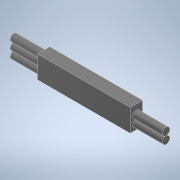
# Autodesk Inventor part: ESC
Saved by Autodesk Inventor 2022 (Build 260153000, 153)
## iProperties
Created: 2022-08-09
Part Number: ESC
Material: Generic
Document SubType Name: Modeling
Designer: Nick
Density: 3.22028 g/cm^3
Appearance: Smooth - Black
Mass: 6.8 g
Surface Area: 17.0549 cm^2
Volume: 2.11162 cm^3
Author: Nick
Autodesk Inventor part; units mm, degrees
ref_plane "YZ Plane" through (0, 0, 0) normal (1, 0, 0) x (0, 1, 0)
ref_plane "XZ Plane" through (0, 0, 0) normal (0, 1, 0) x (-1, 0, 0)
ref_plane "XY Plane" through (0, 0, 0) normal (0, 0, 1) x (1, 0, 0)
sketch "Sketch1" plane through (0, 0, 0) normal (0, 0, 1) x (1, 0, 0)
  line L0 (0, 0) -> (37.5, 0)
  line L1 (37.5, 0) -> (37.5, 9)
  line L2 (37.5, 9) -> (0, 9)
  line L3 (0, 9) -> (0, 0)
  dimension "d0" = 37.5
  dimension "d1" = 9
  constraints: 8 end point, 2 parallel, 1 horizontal, 1 perpendicular
  measures "d0" distance of L1.end L2.end
  measures "d1" distance of L0.end L1.end
extrude "Extrusion1" add sketch "Sketch1" along normal blind 5
sketch "Sketch2" plane through (37.5, 0, 0) normal (1, 0, 0) x (0, 0, -1)
  circle A0 centre (-2.5, 2.3541) radius 1.5
  circle A1 centre (-2.5, 5.3541) radius 1.5
  line L0 (0, 0) -> (-5, 0) projected
  line L1 (0, 9) -> (-5, 9) projected
  point P0 (-2.5, 0)
  dimension "d4" = 3
  constraints: 2 centre point, 2 equal radius, 2 vertical alignment, 1 midpoint
  measures "d4" diameter of A0
extrude "Extrusion2" add sketch "Sketch2" along normal blind 12
sketch "Sketch3" plane through (0, 0, 0) normal (-1, 0, 0) x (0, 0, 1)
  circle A0 centre (2.5, 7.5) radius 1.5
  circle A1 centre (2.5, 4.5) radius 1.5
  circle A2 centre (2.5, 1.5) radius 1.5
  line L0 (0, 9) -> (5, 9) projected
  line L1 (2.5, 7.5) -> (2.5, 9) construction
  line L2 (2.5, 1.5) -> (2.5, 0) construction
  line L3 (0, 0) -> (5, 0) construction
  dimension "d11" = 3
  constraints: 4 end point, 4 equal radius, 3 centre point, 3 vertical alignment, 2 midpoint, 1 collinear, 1 vertical
  measures "d11" diameter of A0
extrude "Extrusion3" add sketch "Sketch3" along normal blind 12
body "Solid1"
